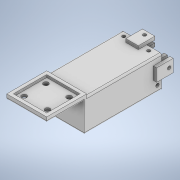
# Autodesk Inventor part: carriageEnd2L
Saved by Autodesk Inventor 2020 (Build 240168000, 168)
## iProperties
Created: 2020-01-10
Part Number: carriageEnd2L
Material: Generic
Document SubType Name: Modeling
Designer: PAB
Density: 1 g/cm^3
Appearance: Default
Author: PAB
Autodesk Inventor part; units mm, degrees
ref_plane "YZ Plane" through (0, 0, 0) normal (1, 0, 0) x (0, 1, 0)
ref_plane "XZ Plane" through (0, 0, 0) normal (0, 1, 0) x (-1, 0, 0)
ref_plane "XY Plane" through (0, 0, 0) normal (0, 0, 1) x (1, 0, 0)
sketch "Sketch1" plane through (0, 0, 0) normal (0, 1, 0) x (-1, 0, 0)
  line L0 (24, 138) -> (-24, 138)
  line L1 (-24, 138) -> (-24, -138)
  line L2 (-24, -138) -> (24, -138)
  line L3 (24, -138) -> (24, 138)
  point P0 (0, 0)
  dimension "d0" = 48
  dimension "d1" = 276
  constraints: 8 end point, 2 parallel, 1 horizontal, 1 perpendicular
  measures "d0" distance of L2.end L1.end
  measures "d1" distance of L1.end L0.end
extrude "Extrusion1" add sketch "Sketch1" along normal blind 3
sketch "Sketch2" plane through (0, 3, 0) normal (0, 1, 0) x (1, 0, 0)
  line L0 (-24, 138) -> (-24, -138) projected
  line L1 (-24, -138) -> (-20, -138)
  line L2 (-20, -138) -> (-20, -90)
  line L3 (-20, -90) -> (-24, -90)
  line L4 (-24, -90) -> (-24, -138)
  line L5 (24, -138) -> (24, 138) projected
  line L6 (-20, -90) -> (24, -90)
  line L7 (24, -90) -> (24, -94)
  line L8 (24, -94) -> (-20, -94)
  line L9 (-20, -94) -> (-20, -90)
  line L10 (-24, -138) -> (24, -138) projected
  line L11 (24, -94) -> (20, -94)
  line L12 (20, -94) -> (20, -138)
  line L13 (20, -138) -> (24, -138)
  line L14 (24, -138) -> (24, -94)
  line L15 (20, -138) -> (-20, -138)
  line L16 (-20, -138) -> (-20, -134)
  line L17 (-20, -134) -> (20, -134)
  line L18 (20, -134) -> (20, -138)
  point P0 (0, 0)
  point P1 (-20, -94)
  dimension "d4" = 4
  dimension "d5" = 48
  dimension "d6" = 4
  dimension "d7" = 4
  dimension "d8" = 4
  constraints: 32 end point, 8 parallel, 4 horizontal, 4 perpendicular, 3 point on line
  measures "d4" distance of L3.end L2.end
  measures "d5" distance of L2.end L1.end
  measures "d6" distance of L6.end L7.end
  measures "d7" distance of L13.end L12.end
  measures "d8" distance of L15.end L16.end
extrude "Extrusion2" add sketch "Sketch2" along normal blind 3 contours L3 L2 L1 L0 | L6 L5 L8 L2 | L2 L17 L12 L10 | L12 L8 L5 L10
mirror "Mirror1" about plane through (0, 0, 0) normal (0, 0, 1) of "Extrusion2"
sketch "Sketch3" plane through (0, 0, 0) normal (0, -1, 0) x (1, 0, 0)
  line L0 (24, -90) -> (-24, -90) projected
  line L1 (24, 138) -> (24, -138) projected
  line L2 (-24, -90) -> (24, -90)
  line L3 (24, -90) -> (24, -93)
  line L4 (24, -93) -> (-24, -93)
  line L5 (-24, -93) -> (-24, -90)
  line L6 (-24, 90) -> (24, 90) projected
  line L7 (24, 90) -> (21, 90)
  line L8 (21, 90) -> (21, -90)
  line L9 (21, -90) -> (24, -90)
  line L10 (24, -90) -> (24, 90)
  line L11 (-24, 90) -> (24, 90)
  line L12 (24, 90) -> (24, 93)
  line L13 (24, 93) -> (-24, 93)
  line L14 (-24, 93) -> (-24, 90)
  point P0 (0, 0)
  dimension "d11" = 3
  dimension "d12" = 3
  dimension "d13" = 3
  constraints: 24 end point, 6 parallel, 3 horizontal, 3 perpendicular, 3 point on line
  measures "d11" distance of L2.end L3.end
  measures "d12" distance of L9.end L8.end
  measures "d13" distance of L12.end L11.end
extrude "Extrusion3" add sketch "Sketch3" along normal blind 35
sketch "Sketch4" plane through (-24, 0, -90) normal (0, 0, 1) x (1, 0, 0)
  line L0 (0, -35) -> (45, -35) projected
  line L1 (45, 0) -> (45, -35) projected
  line L2 (0, -35) -> (45, -35)
  line L3 (45, -35) -> (45, -31)
  line L4 (45, -31) -> (0, -31)
  line L5 (0, -31) -> (0, -35)
  point P0 (24, 0)
  dimension "d16" = 4
  constraints: 8 end point, 2 parallel, 1 horizontal, 1 perpendicular, 1 point on line
  measures "d16" distance of L3.end L2.end
extrude "Extrusion4" add sketch "Sketch4" along normal blind 8
sketch "Sketch5" plane through (-24, -31, -90) normal (0, 1, 0) x (1, 0, 0)
  line L0 (0, -8) -> (45, -8) projected
  line L1 (45, 0) -> (45, -8) projected
  line L2 (0, -8) -> (45, -8)
  line L3 (45, -8) -> (45, -4)
  line L4 (45, -4) -> (0, -4)
  line L5 (0, -4) -> (0, -8)
  point P0 (24, -90)
  dimension "d19" = 4
  constraints: 8 end point, 2 parallel, 1 horizontal, 1 midpoint, 1 perpendicular
  measures "d19" distance of L3.end L2.end
extrude "Extrusion5" add sketch "Sketch5" along normal blind 4
sketch "Sketch6" plane through (0, 0, 0) normal (0, -1, 0) x (1, 0, 0)
  line L0 (21, -86) -> (-24, -86) projected
  line L1 (-24, -82) -> (21, -82)
  line L2 (21, -82) -> (21, -86)
  line L3 (21, -86) -> (-24, -86)
  line L4 (-24, -86) -> (-24, -82)
  point P0 (0, 0)
  dimension "d22" = 4
  constraints: 8 end point, 2 parallel, 1 horizontal, 1 perpendicular
  measures "d22" distance of L1.end L0.start
extrude "Extrusion6" add sketch "Sketch6" along normal blind 4
mirror "Mirror2" about plane through (0, 0, 0) normal (0, 0, 1) of "Extrusion6", "Extrusion5", "Extrusion4"
sketch "Sketch7" plane through (0, 0, 0) normal (0, -1, 0) x (1, 0, 0)
  circle A0 centre (-14, -127) radius 3
  circle A1 centre (14, -127) radius 3
  circle A2 centre (14, -101) radius 3
  circle A3 centre (-14, -101) radius 3
  line L0 (20, -94) -> (20, -134) projected
  line L1 (20, -134) -> (-20, -134) projected
  line L2 (-20, -134) -> (-20, -94) projected
  line L3 (-20, -94) -> (20, -94) projected
  point P0 (0, 0)
  dimension "d25" = 6
  dimension "d26" = 6
  dimension "d27" = 6
  dimension "d28" = 6
  dimension "d101" = 6
  dimension "d102" = 7
  dimension "d103" = 6
  dimension "d104" = 7
  dimension "d105" = 6
  dimension "d106" = 7
  dimension "d107" = 6
  dimension "d108" = 7
  constraints: 4 centre point
  measures "d25" diameter of A0
  measures "d26" diameter of A1
  measures "d27" diameter of A2
  measures "d28" diameter of A3
  measures "d101" distance from line of L0 A1.centre
  measures "d102" distance from line of L1 A1.centre
  measures "d103" distance from line of L2 A0.centre
  measures "d104" distance from line of L1 A0.centre
  measures "d105" distance from line of L2 A3.centre
  measures "d106" distance from line of L3 A3.centre
  measures "d107" distance from line of L0 A2.centre
  measures "d108" distance from line of L3 A2.centre
extrude "Extrusion7" cut sketch "Sketch7" against normal blind 4 contours A0 | A1 | A2 | A3
mirror "Mirror3" about plane through (0, 0, 0) normal (0, 0, 1) of "Extrusion7"
sketch "Sketch12" plane through (0, 0, 0) normal (0, -1, 0) x (1, 0, 0)
  line L0 (21, 82) -> (21, -82) projected
  line L1 (-24, -90) -> (-24, 90) projected
  line L2 (21, 42) -> (-24, 42)
  line L3 (-24, 42) -> (-24, 46)
  line L4 (-24, 46) -> (21, 46)
  line L5 (21, 46) -> (21, 42)
  line L6 (21, 30) -> (-24, 30)
  line L7 (-24, 30) -> (-24, 26)
  line L8 (-24, 26) -> (21, 26)
  line L9 (21, 26) -> (21, 30)
  point P0 (0, 0)
  dimension "d53" = 4
  dimension "d54" = 4
  constraints: 16 end point, 4 parallel, 4 point on line, 2 horizontal, 2 perpendicular
  measures "d53" distance of L2.end L3.end
  measures "d54" distance of L7.end L6.end
extrude "Extrusion12" add sketch "Sketch12" along normal blind 35 contours L0 L2 L1 L4 | L0 L8 L1 L6
sketch "Sketch13" plane through (21, 0, 26) normal (0, 0, -1) x (-1, 0, 0)
  circle A0 centre (30, -20) radius 4
  point P0 (21, 0)
  dimension "d57" = 8
  constraints: 1 centre point
  measures "d57" diameter of A0
extrude "Extrusion13" add sketch "Sketch13" along normal blind 3
sketch "Sketch14" plane through (-24, 0, 46) normal (0, 0, 1) x (1, 0, 0)
  circle A0 centre (15, -20) radius 4 projected
  circle A1 centre (15, -20) radius 4
  point P0 (24, 0)
  dimension "d60" = 8
  constraints: 1 centre point, 1 coincident
  measures "d60" diameter of A1
extrude "Extrusion14" add sketch "Sketch14" along normal blind 3
sketch "Sketch15" plane through (-9, -20, 49) normal (0, 0, 1) x (1, 0, 0)
  circle A0 centre (0, 0) radius 4 projected
  circle A1 centre (0, 0) radius 2
  point P0 (9, 20)
  dimension "d63" = 4
  constraints: 1 centre point, 1 coincident
  measures "d63" diameter of A1
extrude "Extrusion15" cut sketch "Sketch15" against normal blind 30 contours A1
sketch "Sketch16" plane through (21, 0, 26) normal (0, 0, -1) x (-1, 0, 0)
  circle A0 centre (30, -20) radius 4 projected
  circle A1 centre (30, -20) radius 9
  line L0 (45, 0) -> (45, -35) projected
  line L1 (45, -35) -> (40, -35)
  line L2 (40, -35) -> (40, -30)
  line L3 (40, -30) -> (45, -30)
  line L4 (45, -30) -> (45, -35)
  point P0 (21, 0)
  dimension "d66" = 18
  dimension "d67" = 5
  dimension "d68" = 5
  constraints: 8 end point, 2 parallel, 1 centre point, 1 coincident, 1 horizontal, 1 perpendicular
  measures "d66" diameter of A1
  measures "d67" distance of L2.end L3.end
  measures "d68" distance of L1.end L2.end
extrude "Extrusion16" add sketch "Sketch16" against normal blind 20 contours L0 L1 L2 L3
sketch "Sketch17" plane through (21, 0, 26) normal (0, 0, -1) x (-1, 0, 0)
  line L0 (0, -35) -> (0, 0) projected
  line L1 (0, -31) -> (0, 0)
  line L2 (0, 0) -> (31, 0)
  line L3 (0, 0) -> (45, 0) projected
  line L4 (31, 0) -> (0, -31)
  point P0 (21, 0)
  dimension "d71" = 31
  constraints: 6 end point, 2 point on line, 1 collinear
  measures "d71" distance of L0.end L2.end
extrude "Extrusion17" cut sketch "Sketch17" against normal blind 20
sketch "Sketch18" plane through (0, 0, 0) normal (0, -1, 0) x (1, 0, 0)
  line L0 (24, 90) -> (24, -90) projected
  line L1 (-24, -138) -> (-24, -93) projected
  line L2 (24, 0) -> (-24, 0)
  line L3 (-24, 0) -> (-24, -138)
  line L4 (-24, -138) -> (24, -138)
  line L5 (24, -138) -> (24, 0)
  point P0 (0, 0)
  constraints: 8 end point, 2 parallel, 1 horizontal, 1 midpoint, 1 perpendicular
extrude "Extrusion18" cut sketch "Sketch18" along normal mid plane 100
sketch "Sketch19" plane through (0, 0, 0) normal (0, -1, 0) x (1, 0, 0)
  line L0 (-9, 10) -> (6, 10)
  line L1 (6, 10) -> (6, -10)
  line L2 (6, -10) -> (-9, -10)
  line L3 (-9, -10) -> (-9, 10)
  point P0 (0, 0)
  dimension "d76" = 15
  dimension "d77" = 20
  constraints: 8 end point, 2 parallel, 1 horizontal, 1 perpendicular
  measures "d76" distance of L1.end L2.end
  measures "d77" distance of L0.end L1.end
extrude "Extrusion19" add sketch "Sketch19" along normal blind 4 and the other way blind 7
sketch "Sketch20" plane through (21, 0, 86) normal (-1, 0, 0) x (0, 0, 1)
  line L0 (-76, -20) -> (-96, -20)
  line L1 (-96, -20) -> (-96, -5)
  line L2 (-96, -5) -> (-76, -5)
  line L3 (-76, -5) -> (-76, -20)
  point P0 (-86, 0)
  dimension "d82" = 20
  dimension "d83" = 15
  constraints: 8 end point, 2 parallel, 1 horizontal, 1 perpendicular
  measures "d82" distance of L1.end L2.end
  measures "d83" distance of L0.end L1.end
extrude "Extrusion20" add sketch "Sketch20" along normal blind 4 and the other way blind 7
sketch "Sketch21" plane through (0, -4, 0) normal (0, -1, 0) x (1, 0, 0)
  circle A0 centre (-16.5, 5) radius 2
  circle A1 centre (13.5, 5) radius 2
  circle A2 centre (-1.5, -5) radius 2
  point P0 (0, 0)
  dimension "d88" = 4
  dimension "d89" = 4
  dimension "d90" = 4
  constraints: 3 centre point
  measures "d88" diameter of A0
  measures "d89" diameter of A1
  measures "d90" diameter of A2
extrude "Extrusion21" cut sketch "Sketch21" against normal blind 20
sketch "Sketch22" plane through (17, 0, 86) normal (-1, 0, 0) x (0, 0, 1)
  circle A0 centre (-81, -27.5) radius 2
  circle A1 centre (-91, -12.5) radius 2
  point P0 (-86, 0)
  dimension "d93" = 4
  dimension "d94" = 4
  constraints: 2 centre point
  measures "d93" diameter of A0
  measures "d94" diameter of A1
extrude "Extrusion22" cut sketch "Sketch22" against normal blind 20
sketch "Sketch23" plane through (28, -20, -10) normal (0, 0, -1) x (-1, 0, 0)
  line L0 (4, 15) -> (4, 23) projected
  line L1 (7, 0) -> (4, 0)
  line L2 (4, 0) -> (4, 15)
  line L3 (4, 15) -> (7, 15)
  line L4 (7, 15) -> (7, 0)
  line L5 (22, 20) -> (7, 20) projected
  line L6 (22, 20) -> (37, 20)
  line L7 (37, 20) -> (37, 23)
  line L8 (37, 23) -> (22, 23)
  line L9 (22, 23) -> (22, 20)
  point P0 (28, 20)
  constraints: 16 end point, 4 parallel, 2 horizontal, 2 perpendicular
extrude "Extrusion23" cut sketch "Sketch23" against normal blind 10
fillet "Fillet1" radius 2 7 edges at (24, -35, 46.5) (24, 3, 45) (-24, 3, 45) (-24, 0, 115.5) (0, 0, 138) (24, 0, 115.5) (0, -35, 93)
fillet "Fillet2" radius 4 1 edges at (-24, -35, 36)
body "Solid1"
